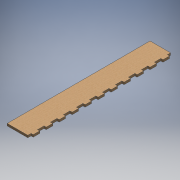
# Autodesk Inventor part: BearingMotorColumnSupport
Saved by Autodesk Inventor 2016 (Build 200138000, 138)
## iProperties
Created: 2015-11-25
Part Number: BearingMotorColumnSupport
Material: MDF Medium Density Fiberboard
Document SubType Name: Modeling
Designer: momem
Density: 0.8 g/cm^3
Appearance: Cardboard - Corrugated
Author: momem
Autodesk Inventor part; units mm, degrees
ref_plane "YZ Plane" through (0, 0, 0) normal (1, 0, 0) x (0, 1, 0)
ref_plane "XZ Plane" through (0, 0, 0) normal (0, 1, 0) x (-1, 0, 0)
ref_plane "XY Plane" through (0, 0, 0) normal (0, 0, 1) x (1, 0, 0)
sketch "Sketch2" plane through (0, 0, 0) normal (0, 0, 1) x (1, 0, 0)
  line L0 (60, 28.4382) -> (66.39, 28.4382)
  line L1 (66.39, 28.4382) -> (66.39, 9.4794)
  line L2 (66.39, 9.4794) -> (60, 9.4794)
  line L3 (60, 66.3559) -> (66.39, 66.3559)
  line L4 (66.39, 66.3559) -> (66.39, 47.3971)
  line L5 (66.39, 47.3971) -> (60, 47.3971)
  line L6 (60, 104.2736) -> (66.39, 104.2736)
  line L7 (66.39, 104.2736) -> (66.39, 85.3147)
  line L8 (66.39, 85.3147) -> (60, 85.3147)
  line L9 (60, 142.1912) -> (66.39, 142.1912)
  line L10 (66.39, 142.1912) -> (66.39, 123.2324)
  line L11 (66.39, 123.2324) -> (60, 123.2324)
  line L12 (60, 180.1089) -> (66.39, 180.1089)
  line L13 (66.39, 180.1089) -> (66.39, 161.15)
  line L14 (66.39, 161.15) -> (60, 161.15)
  line L15 (60, 218.0265) -> (66.39, 218.0265)
  line L16 (66.39, 218.0265) -> (66.39, 199.0677)
  line L17 (66.39, 199.0677) -> (60, 199.0677)
  line L18 (60, 255.9442) -> (66.39, 255.9442)
  line L19 (66.39, 255.9442) -> (66.39, 236.9854)
  line L20 (66.39, 236.9854) -> (60, 236.9854)
  line L21 (60, 293.8619) -> (66.39, 293.8619)
  line L22 (66.39, 293.8619) -> (66.39, 274.903)
  line L23 (66.39, 274.903) -> (60, 274.903)
  line L24 (60, 331.7795) -> (66.39, 331.7795)
  line L25 (66.39, 331.7795) -> (66.39, 312.8207)
  line L26 (66.39, 312.8207) -> (60, 312.8207)
  line L27 (60, 369.6972) -> (66.39, 369.6972)
  line L28 (66.39, 369.6972) -> (66.39, 350.7383)
  line L29 (66.39, 350.7383) -> (60, 350.7383)
  line L30 (60, 407.6148) -> (66.39, 407.6148)
  line L31 (66.39, 407.6148) -> (66.39, 388.656)
  line L32 (66.39, 388.656) -> (60, 388.656)
  line L33 (60, 407.6148) -> (60, 417.0942)
  line L34 (60, 417.0942) -> (0, 417.0942)
  line L35 (0, 417.0942) -> (0, 0)
  line L36 (0, 0) -> (60, 0)
  line L37 (60, 0) -> (60, 9.4794)
  line L38 (60, 28.4382) -> (60, 47.3971)
  line L39 (60, 66.3559) -> (60, 85.3147)
  line L40 (60, 104.2736) -> (60, 123.2324)
  line L41 (60, 142.1912) -> (60, 161.15)
  line L42 (60, 180.1089) -> (60, 199.0677)
  line L43 (60, 388.656) -> (60, 369.6972)
  line L44 (60, 350.7383) -> (60, 331.7795)
  line L45 (60, 312.8207) -> (60, 293.8619)
  line L46 (60, 274.903) -> (60, 255.9442)
  line L47 (60, 236.9854) -> (60, 218.0265)
  line L48 (66.39, 18.9588) -> (0, 18.9588) construction
  dimension "d56" = 18.9588
  dimension "d58" = 6.39
  dimension "d72" = 37.9177
  dimension "d77" = 60
  dimension "d78" = 9.4794
  dimension "d79" = 9.4794
  dimension "d80" = 417.0942
  constraints: 98 end point, 8 equal length, 6 perpendicular, 5 vertical, 2 point on line, 1 collinear, 1 horizontal, 1 midpoint, 70 other
  measures "d56" distance between parallel lines of L2 L0
  measures "d58" distance of L0.start L0.end
  measures "d72" distance of L0.start L3.start
  measures "d77" distance of L35.end L36.end
  measures "d78" distance of L30.start L33.end
  measures "d79" distance of L36.end L2.end
  measures "d80" distance of L34.end L35.end
extrude "Extrusion5" add sketch "Sketch2" along normal blind 6.39
equation "\"d56\" = 0.25 * DiskGap"
equation "\"d58\" = WoodThickness"
equation "\"d72\" = 0.5 * DiskGap"
equation "\"d78\" = 0.125 * DiskGap"
equation "\"d79\" = 0.125 * DiskGap"
equation "\"d94\" = WoodThickness"
equation "\"MotorWidth\" = 37"
equation "\"SupportClearance\" = 5"
equation "\"MotorShaftWidth\" = 12"
equation "\"CouplingWidth\" = 9.525"
equation "\"CouplingDiameter\" = 22.098"
equation "\"DiskGap\" = 75.835317"
equation "\"WoodThickness\" = 6.39"
body "Solid4"
